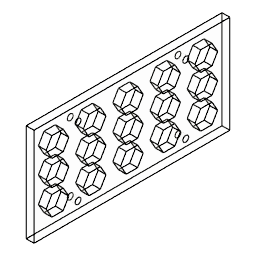
Lado 2 (Autodesk Fusion 360 design; units mm, degrees)
Autodesk Fusion 360 part; units mm, degrees
note: some values were not read from the file. Set by a fixed rule: which sketch regions a step uses.
sketch "Boceto1" plane through (0, 0, 0) normal (0, 1, 0) x (1, 0, 0)
  line L0 (0, 0) -> (4, 0)
  line L1 (4, 0) -> (4, 100)
  line L2 (4, 100) -> (0, 100)
  line L3 (0, 100) -> (0, 0)
  dimension "d1" = 4
  dimension "d2" = 100
  constraint coincident L0.start L3.end
  constraint horizontal L0
  constraint perpendicular L0 L1
  constraint perpendicular L1 L2
  constraint perpendicular L0 L3
  measures "d1" distance of L0.start L0.end
  measures "d2" distance of L0.end L1.end
extrude "Extruir1" add sketch "Boceto1" along normal blind 50
sketch "Boceto2" plane through (4, 0, 0) normal (1, 0, 0) x (0, 0, -1)
  line L0 (0, 0) -> (100, 0)
  line L1 (100, 0) -> (100, 50)
  line L2 (100, 50) -> (0, 50)
  line L3 (0, 50) -> (0, 0)
  line L4 (0, 0) -> (0, 7.5)
  line L5 (0, 7.5) -> (22.5, 7.5)
  line L6 (22.5, 7.5) -> (77.5, 7.5)
  line L7 (77.5, 7.5) -> (77.5, 42.5)
  line L8 (77.5, 42.5) -> (22.5, 42.5)
  circle A0 centre (22.5, 42.5) radius 1.5
  circle A1 centre (77.5, 42.5) radius 1.5
  circle A2 centre (22.5, 7.5) radius 1.5
  circle A3 centre (77.5, 7.5) radius 1.5
  line L9 (0, 50) -> (4, 50)
  line L10 (4, 50) -> (4, 46)
  line L11 (4, 46) -> (96, 46)
  line L12 (96, 46) -> (96, 4)
  line L13 (96, 4) -> (4, 4)
  line L14 (4, 4) -> (4, 46)
  line L15 (50, 46) -> (50, 25)
  line L16 (47.1132, 30) -> (44.2265, 25)
  line L17 (44.2265, 25) -> (47.1132, 20)
  line L18 (47.1132, 20) -> (52.8868, 20)
  line L19 (52.8868, 20) -> (55.7735, 25)
  line L20 (55.7735, 25) -> (52.8868, 30)
  line L21 (52.8868, 30) -> (47.1132, 30)
  line L22 (9.1132, 30) -> (6.2265, 25)
  line L23 (9.1132, 20) -> (14.8868, 20)
  line L24 (14.8868, 20) -> (17.7735, 25)
  line L25 (6.2265, 25) -> (9.1132, 20)
  line L26 (17.7735, 25) -> (14.8868, 30)
  line L27 (14.8868, 30) -> (9.1132, 30)
  line L28 (28.1132, 30) -> (25.2265, 25)
  line L29 (28.1132, 20) -> (33.8868, 20)
  line L30 (33.8868, 20) -> (36.7735, 25)
  line L31 (25.2265, 25) -> (28.1132, 20)
  line L32 (36.7735, 25) -> (33.8868, 30)
  line L33 (33.8868, 30) -> (28.1132, 30)
  line L34 (66.1132, 30) -> (63.2265, 25)
  line L35 (66.1132, 20) -> (71.8868, 20)
  line L36 (71.8868, 20) -> (74.7735, 25)
  line L37 (63.2265, 25) -> (66.1132, 20)
  line L38 (74.7735, 25) -> (71.8868, 30)
  line L39 (71.8868, 30) -> (66.1132, 30)
  line L40 (85.1132, 30) -> (82.2265, 25)
  line L41 (85.1132, 20) -> (90.8868, 20)
  line L42 (90.8868, 20) -> (93.7735, 25)
  line L43 (82.2265, 25) -> (85.1132, 20)
  line L44 (93.7735, 25) -> (90.8868, 30)
  line L45 (90.8868, 30) -> (85.1132, 30)
  line L46 (17.7735, 12) -> (14.8868, 17)
  line L47 (85.1132, 17) -> (82.2265, 12)
  line L48 (14.8868, 17) -> (9.1132, 17)
  line L49 (90.8868, 7) -> (93.7735, 12)
  line L50 (47.1132, 7) -> (52.8868, 7)
  line L51 (28.1132, 17) -> (25.2265, 12)
  line L52 (47.1132, 17) -> (44.2265, 12)
  line L53 (85.1132, 7) -> (90.8868, 7)
  line L54 (52.8868, 7) -> (55.7735, 12)
  line L55 (63.2265, 12) -> (66.1132, 7)
  line L56 (9.1132, 7) -> (14.8868, 7)
  line L57 (14.8868, 7) -> (17.7735, 12)
  line L58 (52.8868, 17) -> (47.1132, 17)
  line L59 (74.7735, 12) -> (71.8868, 17)
  line L60 (28.1132, 7) -> (33.8868, 7)
  line L61 (36.7735, 12) -> (33.8868, 17)
  line L62 (82.2265, 12) -> (85.1132, 7)
  line L63 (71.8868, 17) -> (66.1132, 17)
  line L64 (33.8868, 17) -> (28.1132, 17)
  line L65 (93.7735, 12) -> (90.8868, 17)
  line L66 (9.1132, 17) -> (6.2265, 12)
  line L67 (33.8868, 7) -> (36.7735, 12)
  line L68 (25.2265, 12) -> (28.1132, 7)
  line L69 (71.8868, 7) -> (74.7735, 12)
  line L70 (55.7735, 12) -> (52.8868, 17)
  line L71 (6.2265, 12) -> (9.1132, 7)
  line L72 (66.1132, 7) -> (71.8868, 7)
  line L73 (66.1132, 17) -> (63.2265, 12)
  line L74 (44.2265, 12) -> (47.1132, 7)
  line L75 (90.8868, 17) -> (85.1132, 17)
  line L76 (17.7735, 38) -> (14.8868, 43)
  line L77 (85.1132, 43) -> (82.2265, 38)
  line L78 (14.8868, 43) -> (9.1132, 43)
  line L79 (90.8868, 33) -> (93.7735, 38)
  line L80 (47.1132, 33) -> (52.8868, 33)
  line L81 (28.1132, 43) -> (25.2265, 38)
  line L82 (47.1132, 43) -> (44.2265, 38)
  line L83 (85.1132, 33) -> (90.8868, 33)
  line L84 (52.8868, 33) -> (55.7735, 38)
  line L85 (63.2265, 38) -> (66.1132, 33)
  line L86 (9.1132, 33) -> (14.8868, 33)
  line L87 (14.8868, 33) -> (17.7735, 38)
  line L88 (52.8868, 43) -> (47.1132, 43)
  line L89 (74.7735, 38) -> (71.8868, 43)
  line L90 (28.1132, 33) -> (33.8868, 33)
  line L91 (36.7735, 38) -> (33.8868, 43)
  line L92 (82.2265, 38) -> (85.1132, 33)
  line L93 (71.8868, 43) -> (66.1132, 43)
  line L94 (33.8868, 43) -> (28.1132, 43)
  line L95 (93.7735, 38) -> (90.8868, 43)
  line L96 (9.1132, 43) -> (6.2265, 38)
  line L97 (33.8868, 33) -> (36.7735, 38)
  line L98 (25.2265, 38) -> (28.1132, 33)
  line L99 (71.8868, 33) -> (74.7735, 38)
  line L100 (55.7735, 38) -> (52.8868, 43)
  line L101 (6.2265, 38) -> (9.1132, 33)
  line L102 (66.1132, 33) -> (71.8868, 33)
  line L103 (66.1132, 43) -> (63.2265, 38)
  line L104 (44.2265, 38) -> (47.1132, 33)
  line L105 (90.8868, 43) -> (85.1132, 43)
  point P0 (50, 25)
  point P1 (12, 25)
  point P2 (12, 25)
  point P3 (31, 25)
  point P4 (31, 25)
  point P5 (69, 25)
  point P6 (69, 25)
  point P7 (88, 25)
  point P8 (88, 25)
  point P9 (12, 12)
  point P10 (50, 12)
  point P11 (69, 12)
  point P12 (31, 12)
  point P13 (88, 12)
  point P14 (50, 12)
  point P15 (31, 12)
  point P16 (88, 12)
  point P17 (69, 12)
  point P18 (12, 12)
  point P19 (12, 38)
  point P20 (50, 38)
  point P21 (69, 38)
  point P22 (31, 38)
  point P23 (88, 38)
  point P24 (50, 38)
  point P25 (31, 38)
  point P26 (88, 38)
  point P27 (69, 38)
  point P28 (12, 38)
  dimension "d5" = 7.5
  dimension "d6" = 22.5
  dimension "d7" = 55
  dimension "d8" = 35
  dimension "d9" = 3
  dimension "d10" = 3
  dimension "d11" = 3
  dimension "d12" = 3
  dimension "d13" = 4
  dimension "d14" = 4
  dimension "d15" = 92
  dimension "d16" = 42
  dimension "d17" = 5
  dimension "d20" = 38
  dimension "d21" = 0
  dimension "d24" = 0
  dimension "d25" = 13
  constraint coincident L0.start L3.end
  constraint coincident L3 L4.end
  constraint perpendicular L3 L5
  constraint perpendicular L1 L6
  constraint perpendicular L2 L7
  constraint perpendicular L7 L8
  constraint coincident L8.end A0.centre
  constraint coincident L7.end L8.start
  constraint coincident L5.end L6.start
  constraint coincident L6.end L7.start
  constraint coincident L2.end L3.start
  constraint perpendicular L3 L9
  constraint perpendicular L2 L10
  constraint perpendicular L1 L11
  constraint perpendicular L0 L12
  constraint perpendicular L10 L13
  constraint perpendicular L13 L14
  constraint midpoint L11 L15.start
  constraint perpendicular L6 L15
  constraint coincident P0 L15.end
  measures "d5" distance of L0.start L4.end
  measures "d6" distance of L4.end L5.end
  measures "d7" distance of L5.end L6.end
  measures "d8" distance of L6.end L7.end
  measures "d9" diameter of A0
  measures "d10" diameter of A1
  measures "d11" diameter of A2
  measures "d12" diameter of A3
  measures "d13" distance of L2.end L9.end
  measures "d14" distance of L9.end L10.end
  measures "d15" distance of L10.end L11.end
  measures "d16" distance of L11.end L12.end
  measures "d17" distance of P0 L21
extrude "Extruir2" cut sketch "Boceto2" against normal blind 13 contours L5 L46 L48 L57 L66 L71 | L5 L56 L57 L71 | L5 L6 A2 | L5 L6 A2 | L8 L15 L88 L100 | L8 L15 L82 L88 | L8 L15 L80 L82 L104 | L8 L15 L80 L84 L100 | L6 L51 L61 L64 L67 L68 | L6 L60 L67 L68 | L8 L89 L93 L103 | L8 L85 L89 L99 L102 L103 | L6 L52 L54 L58 L70 L74 | L6 L50 L54 L74 | L7 L8 A1 | L7 L8 A1 | L6 L55 L59 L63 L69 L73 | L6 L55 L69 L72 | L6 L7 A3 | L6 L7 A3 | L8 L81 L90 L91 L97 L98 | L8 L81 L91 L94 | A0 | L16 L17 L18 L19 L20 L21 | L22 L23 L24 L25 L26 L27 | L28 L29 L30 L31 L32 L33 | L34 L35 L36 L37 L38 L39 | L40 L41 L42 L43 L44 L45 | L47 L49 L53 L62 L65 L75 | L76 L78 L86 L87 L96 L101 | L77 L79 L83 L92 L95 L105
sketch "Boceto3" plane through (4, 0, 0) normal (1, 0, 0) x (0, 0, -1)
  line L0 (52.8868, 7) -> (47.1132, 7)
  line L1 (47.1132, 7) -> (44.2265, 12)
  line L2 (44.2265, 12) -> (47.1132, 17)
  line L3 (47.1132, 17) -> (52.8868, 17)
  line L4 (52.8868, 17) -> (55.7735, 12)
  line L5 (55.7735, 12) -> (52.8868, 7)
  line L6 (14.8868, 33) -> (9.1132, 33)
  line L7 (9.1132, 33) -> (6.2265, 38)
  line L8 (6.2265, 38) -> (9.1132, 43)
  line L9 (9.1132, 43) -> (14.8868, 43)
  line L10 (14.8868, 43) -> (17.7735, 38)
  line L11 (17.7735, 38) -> (14.8868, 33)
  line L12 (63.2265, 25) -> (66.1132, 30)
  line L13 (66.1132, 30) -> (71.8868, 30)
  line L14 (71.8868, 30) -> (74.7735, 25)
  line L15 (74.7735, 25) -> (71.8868, 20)
  line L16 (71.8868, 20) -> (66.1132, 20)
  line L17 (66.1132, 20) -> (63.2265, 25)
  circle A0 centre (77.5, 42.5) radius 1.5
  circle A1 centre (22.5, 42.5) radius 1.5
  line L18 (66.1132, 33) -> (63.2265, 38)
  line L19 (63.2265, 38) -> (66.1132, 43)
  line L20 (66.1132, 43) -> (71.8868, 43)
  line L21 (71.8868, 43) -> (74.7735, 38)
  line L22 (74.7735, 38) -> (71.8868, 33)
  line L23 (71.8868, 33) -> (66.1132, 33)
  line L24 (82.2265, 12) -> (85.1132, 17)
  line L25 (85.1132, 17) -> (90.8868, 17)
  line L26 (90.8868, 17) -> (93.7735, 12)
  line L27 (93.7735, 12) -> (90.8868, 7)
  line L28 (90.8868, 7) -> (85.1132, 7)
  line L29 (85.1132, 7) -> (82.2265, 12)
  line L30 (6.2265, 25) -> (9.1132, 30)
  line L31 (9.1132, 30) -> (14.8868, 30)
  line L32 (14.8868, 30) -> (17.7735, 25)
  line L33 (17.7735, 25) -> (14.8868, 20)
  line L34 (14.8868, 20) -> (9.1132, 20)
  line L35 (9.1132, 20) -> (6.2265, 25)
  line L36 (33.8868, 7) -> (28.1132, 7)
  line L37 (28.1132, 7) -> (25.2265, 12)
  line L38 (25.2265, 12) -> (28.1132, 17)
  line L39 (28.1132, 17) -> (33.8868, 17)
  line L40 (33.8868, 17) -> (36.7735, 12)
  line L41 (36.7735, 12) -> (33.8868, 7)
  line L42 (66.1132, 7) -> (63.2265, 12)
  line L43 (63.2265, 12) -> (66.1132, 17)
  line L44 (66.1132, 17) -> (71.8868, 17)
  line L45 (71.8868, 17) -> (74.7735, 12)
  line L46 (74.7735, 12) -> (71.8868, 7)
  line L47 (71.8868, 7) -> (66.1132, 7)
  line L48 (14.8868, 7) -> (9.1132, 7)
  line L49 (9.1132, 7) -> (6.2265, 12)
  line L50 (6.2265, 12) -> (9.1132, 17)
  line L51 (9.1132, 17) -> (14.8868, 17)
  line L52 (14.8868, 17) -> (17.7735, 12)
  line L53 (17.7735, 12) -> (14.8868, 7)
  line L54 (44.2265, 25) -> (47.1132, 30)
  line L55 (47.1132, 30) -> (52.8868, 30)
  line L56 (52.8868, 30) -> (55.7735, 25)
  line L57 (55.7735, 25) -> (52.8868, 20)
  line L58 (52.8868, 20) -> (47.1132, 20)
  line L59 (47.1132, 20) -> (44.2265, 25)
  line L60 (82.2265, 38) -> (85.1132, 43)
  line L61 (85.1132, 43) -> (90.8868, 43)
  line L62 (90.8868, 43) -> (93.7735, 38)
  line L63 (93.7735, 38) -> (90.8868, 33)
  line L64 (90.8868, 33) -> (85.1132, 33)
  line L65 (85.1132, 33) -> (82.2265, 38)
  line L66 (33.8868, 33) -> (28.1132, 33)
  line L67 (28.1132, 33) -> (25.2265, 38)
  line L68 (25.2265, 38) -> (28.1132, 43)
  line L69 (28.1132, 43) -> (33.8868, 43)
  line L70 (33.8868, 43) -> (36.7735, 38)
  line L71 (36.7735, 38) -> (33.8868, 33)
  line L72 (52.8868, 33) -> (47.1132, 33)
  line L73 (47.1132, 33) -> (44.2265, 38)
  line L74 (44.2265, 38) -> (47.1132, 43)
  line L75 (47.1132, 43) -> (52.8868, 43)
  line L76 (52.8868, 43) -> (55.7735, 38)
  line L77 (55.7735, 38) -> (52.8868, 33)
  line L78 (82.2265, 25) -> (85.1132, 30)
  line L79 (85.1132, 30) -> (90.8868, 30)
  line L80 (90.8868, 30) -> (93.7735, 25)
  line L81 (93.7735, 25) -> (90.8868, 20)
  line L82 (90.8868, 20) -> (85.1132, 20)
  line L83 (85.1132, 20) -> (82.2265, 25)
  line L84 (25.2265, 25) -> (28.1132, 30)
  line L85 (28.1132, 30) -> (33.8868, 30)
  line L86 (33.8868, 30) -> (36.7735, 25)
  line L87 (36.7735, 25) -> (33.8868, 20)
  line L88 (33.8868, 20) -> (28.1132, 20)
  line L89 (28.1132, 20) -> (25.2265, 25)
  circle A2 centre (22.5, 7.5) radius 1.5
  circle A3 centre (77.5, 7.5) radius 1.5
  line L90 (0, 0) -> (100, 0)
  line L91 (100, 0) -> (100, 50)
  line L92 (100, 50) -> (0, 50)
  line L93 (0, 50) -> (0, 0)
